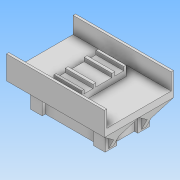
# Autodesk Inventor part: Viaduct_HorizontalSingle
Saved by Autodesk Inventor 2021 (Build 250183000, 183)
## iProperties
Created: 2021-03-16
Part Number: Viaduct_HorizontalSingle
Material: 一般
Document SubType Name: Modeling
Designer: kumagai
Density: 1 g/cm^3
Appearance: 既定
Author: kumagai
Autodesk Inventor part; units mm, degrees
ref_plane "YZ Plane" through (0, 0, 0) normal (1, 0, 0) x (0, 1, 0)
ref_plane "XY Plane" through (0, 0, 0) normal (0, 0, 1) x (1, 0, 0)
sketch "スケッチ1" plane through (0, 0, 0) normal (1, 0, 0) x (0, 1, 0)
  line L0 (0, 41.3) -> (0, -41.3) projected
  line L1 (-39, 0) -> (17, 0) projected
  line L2 (-5.2, 19) -> (3.2, 19)
  line L3 (3.2, 19) -> (3.2, 17)
  line L4 (3.2, 17) -> (0, 17)
  line L5 (0, 17) -> (0, 9.3)
  line L6 (0, 9.3) -> (3.2, 9.3)
  line L7 (3.2, 9.3) -> (3.2, 6.9)
  line L8 (3.2, 6.9) -> (0, 6.9)
  line L9 (0, 6.9) -> (0, -6.9)
  line L10 (0, -6.9) -> (3.2, -6.9)
  line L11 (3.2, -6.9) -> (3.2, -9.3)
  line L12 (3.2, -9.3) -> (0, -9.3)
  line L13 (0, -9.3) -> (0, -17)
  line L14 (0, -17) -> (3.2, -17)
  line L15 (3.2, -17) -> (3.2, -19)
  line L16 (3.2, -19) -> (-5.2, -19)
  line L17 (-5.2, -19) -> (-5.2, 19)
  line L18 (-5.2, 27.5) -> (-5.2, -27.5)
  line L19 (-5.2, -27.5) -> (9, -27.5)
  line L20 (9, -27.5) -> (9, -29.5)
  line L21 (9, -29.5) -> (-11, -29.5)
  line L22 (-11, -29.5) -> (-11, 29.5)
  line L23 (-11, 29.5) -> (9, 29.5)
  line L24 (9, 29.5) -> (9, 27.5)
  line L25 (9, 27.5) -> (-5.2, 27.5)
  line L26 (-11, 29.5) -> (-22.3278, 16)
  line L27 (-22.3278, 16) -> (-31, 16)
  line L28 (-31, 16) -> (-31, 12)
  line L29 (-31, 12) -> (-21.0692, 12)
  line L30 (-21.0692, 12) -> (-11, 0)
  line L31 (-11, 0) -> (-21.0692, -12)
  line L32 (-21.0692, -12) -> (-31, -12)
  line L33 (-31, -12) -> (-31, -16)
  line L34 (-31, -16) -> (-22.3278, -16)
  line L35 (-22.3278, -16) -> (-11, -29.5)
  point P0 (0, 0)
  dimension "d0" = 38
  dimension "d1" = 18.6
  dimension "d2" = 2
  dimension "d3" = 2.4
  dimension "d4" = 3.2
  dimension "d5" = 8.4
  dimension "d6" = 59
  dimension "d7" = 2
  dimension "d8" = 20
  dimension "d9" = 5.8
  dimension "d10" = 5.8
  dimension "d11" = 40
  dimension "d12" = 40
  dimension "d13" = 32
  dimension "d14" = 4
  dimension "d15" = 20
  constraints: 68 end point, 9 point on line, 2 horizontal, 2 vertical, 1 collinear, 1 midpoint, 17 other
  measures "d0" distance between parallel lines of L16 L2
  measures "d1" distance between parallel lines of L12 L6
  measures "d2" distance between parallel lines of L2 L4
  measures "d3" distance between parallel lines of L6 L8
  measures "d4" distance between parallel lines of L13 L15
  measures "d5" distance between parallel lines of L17 L15
  measures "d6" distance between parallel lines of L21 L23
  measures "d7" distance between parallel lines of L23 L25
  measures "d8" distance between parallel lines of L22 L24
  measures "d9" distance between parallel lines of L24 L3
  measures "d10" distance between parallel lines of L22 L18
  measures "d11" angle of L22 L26
  measures "d12" angle of L22 L30
  measures "d13" distance between parallel lines of L34 L27
  measures "d14" distance between parallel lines of L27 L29
  measures "d15" distance between parallel lines of L22 L33
extrude "押し出し1" add sketch "スケッチ1" along normal mid plane 23.75 contours L0 L1 L17 L2 | L0 L2 L3 L4 | L6 L7 L8 L0 | L0 L16 L17 L1 | L10 L11 L12 L0 | L0 L14 L15 L16
extrude "押し出し2" add sketch "スケッチ1" along normal mid plane 83.75 contours L25 L18 L17 L1 L22 L23 L0 | L0 L23 L24 L25 | L17 L18 L19 L0 L21 L22 L1 | L22 L30 L29 L28 L27 L26 | L22 L35 L34 L33 L32 L31 | L0 L19 L20 L21
ref_plane "作業平面1" through (0, -32.2, 0) normal (0, 1, 0) x (-1, 0, 0)
sketch "スケッチ2" plane through (0, -32.2, 0) normal (0, 1, 0) x (-1, 0, 0)
  line L0 (0, -41.3) -> (0, 41.3) projected
  line L1 (-58.625, 0) -> (58.625, 0) projected
  line L2 (31.875, -19) -> (21.875, -19)
  line L3 (21.875, -19) -> (21.875, -9)
  line L4 (21.875, -9) -> (31.875, -9)
  line L5 (31.875, -9) -> (31.875, -19)
  line L6 (-21.875, -19) -> (-31.875, -19)
  line L7 (-31.875, -19) -> (-31.875, -9)
  line L8 (-31.875, -9) -> (-21.875, -9)
  line L9 (-21.875, -9) -> (-21.875, -19)
  line L10 (31.875, 9) -> (21.875, 9)
  line L11 (21.875, 9) -> (21.875, 19)
  line L12 (21.875, 19) -> (31.875, 19)
  line L13 (31.875, 19) -> (31.875, 9)
  line L14 (-21.875, 9) -> (-31.875, 9)
  line L15 (-31.875, 9) -> (-31.875, 19)
  line L16 (-31.875, 19) -> (-21.875, 19)
  line L17 (-21.875, 19) -> (-21.875, 9)
  line L18 (-21.875, 16.2551) -> (21.875, 16.2551)
  line L19 (21.875, 16.2551) -> (21.875, 12)
  line L20 (21.875, 12) -> (-21.875, 12)
  line L21 (-21.875, 12) -> (-21.875, 16.2551)
  line L22 (21.875, -12) -> (-21.875, -12)
  line L23 (-21.875, -12) -> (-21.875, -16.2551)
  line L24 (-21.875, -16.2551) -> (21.875, -16.2551)
  line L25 (21.875, -16.2551) -> (21.875, -12)
  line L26 (-28.875, 9) -> (-24.875, 9)
  line L27 (-24.875, 9) -> (-24.875, -9)
  line L28 (-24.875, -9) -> (-28.875, -9)
  line L29 (-28.875, -9) -> (-28.875, 9)
  line L30 (24.875, 9) -> (28.875, 9)
  line L31 (28.875, 9) -> (28.875, -9)
  line L32 (28.875, -9) -> (24.875, -9)
  line L33 (24.875, -9) -> (24.875, 9)
  point P0 (0, 0)
  dimension "d21" = 38
  dimension "d23" = 53.75
  dimension "d24" = 10
  dimension "d25" = 10
  dimension "d28" = 3
  dimension "d29" = 3
  dimension "d30" = 3
  dimension "d31" = 2.7449
  constraints: 64 end point, 11 point on line, 8 collinear, 8 other
  measures "d21" distance between parallel lines of L16 L6
  measures "d23" distance between parallel lines of L9 L5
  measures "d24" distance between parallel lines of L5 L3
  measures "d25" distance between parallel lines of L4 L2
  measures "d28" distance between parallel lines of L15 L29
  measures "d29" distance between parallel lines of L17 L27
  measures "d30" distance between parallel lines of L14 L20
  measures "d31" distance between parallel lines of L18 L16
extrude "押し出し3" add sketch "スケッチ2" along normal up to next contours L24 L9 L22 L0 | L0 L22 L3 L24 | L9 L6 L7 L8 | L3 L4 L5 L2 | L20 L17 L18 L0 | L0 L18 L11 L20 | L27 L8 L29 L1 | L1 L29 L14 L27 | L33 L10 L31 L1 | L1 L31 L4 L33 | L11 L12 L13 L10 | L17 L14 L15 L16
sketch "スケッチ3" plane through (0, 0, 0) normal (0, 0, 1) x (1, 0, 0)
  line L0 (-41.875, -11) -> (-31.875, -31)
  line L1 (-31.875, -31) -> (-41.875, -31)
  line L2 (-41.875, -31) -> (-41.875, -11)
  line L3 (0, 17.24) -> (0, -40.44) projected
  line L4 (41.875, -11) -> (31.875, -31)
  line L5 (31.875, -31) -> (41.875, -31)
  line L6 (41.875, -31) -> (41.875, -11)
  point P0 (0, 0)
  constraints: 12 end point, 3 symmetric about line, 1 horizontal, 1 vertical
extrude "押し出し4" cut sketch "スケッチ3" against normal through all both and the other way through all
equation "\"d0\" = RailWidth"
equation "\"d1\" = InsideWidth"
equation "\"d2\" = OuterWall"
equation "\"d3\" = InnerWall"
equation "\"d4\" = RailDepth"
equation "\"d5\" = RailHeight"
equation "\"d9\" = d10"
equation "\"d16\" = Length - 2 * ConnectorLength"
equation "\"d21\" = RailWidth"
equation "\"d23\" = Length"
equation "\"d29\" = d28"
equation "\"d30\" = d28"
equation "\"Length\" = 0.25 * StraightLength"
equation "\"RailWidth\" = 38"
equation "\"InsideWidth\" = 18.6"
equation "\"OuterWall\" = 2"
equation "\"InnerWall\" = 2.4"
equation "\"RailDepth\" = 3.2"
equation "\"RailHeight\" = 8.4"
equation "\"ConnectorLength\" = 15"
equation "\"StraightLength\" = 215"
